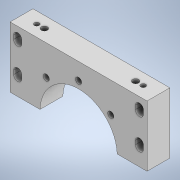
# Autodesk Inventor part: ShooterSeperableClampA
Saved by Autodesk Inventor 2020 (Build 240168000, 168)
## iProperties
Created: 2020-01-29
Part Number: ShooterSeperableClampA
Material: Generic
Document SubType Name: Modeling
Designer: srini
Density: 1 g/cm^3
Appearance: Default
Author: srini
Autodesk Inventor part; units mm, degrees
ref_plane "YZ Plane" through (0, 0, 0) normal (1, 0, 0) x (0, 1, 0)
ref_plane "XZ Plane" through (0, 0, 0) normal (0, 1, 0) x (-1, 0, 0)
ref_plane "XY Plane" through (0, 0, 0) normal (0, 0, 1) x (1, 0, 0)
sketch "Sketch1" plane through (0, 0, 0) normal (0, 0, 1) x (1, 0, 0)
  line L0 (57.15, -25.4) -> (-57.15, -25.4)
  line L1 (-57.15, -25.4) -> (-57.15, 25.4)
  line L2 (-57.15, 25.4) -> (57.15, 25.4)
  line L3 (57.15, 25.4) -> (57.15, -25.4)
  line L4 (57.15, -25.4) -> (-57.15, 25.4) construction
  line L5 (-57.15, -25.4) -> (57.15, 25.4) construction
  point P0 (0, 0)
  point P1 (0, 0)
  point P2 (0, 0)
  dimension "d0" = 114.3
  dimension "d1" = 50.8
  constraints: 12 end point, 3 midpoint, 2 parallel, 1 coincident, 1 horizontal, 1 perpendicular
  measures "d0" distance of L1.end L2.end
  measures "d1" distance of L0.end L1.end
extrude "Extrusion1" add sketch "Sketch1" along normal blind 19.05
sketch "Sketch2" plane through (0, 0, 19.05) normal (0, 0, 1) x (1, 0, 0)
  circle A0 centre (0, -26.67) radius 32.258
  line L0 (-57.15, -25.4) -> (57.15, -25.4) projected
  point P0 (0, 0)
  dimension "d4" = 64.516
  dimension "d6" = 1.27
  constraints: 1 centre point, 1 vertical alignment
  measures "d4" diameter of A0
  measures "d6" distance from line of L0 A0.centre
extrude "Extrusion2" cut sketch "Sketch2" against normal through all
sketch "Sketch3" plane through (0, 0, 19.05) normal (0, 0, 1) x (1, 0, 0)
  line L0 (57.15, 25.4) -> (-57.15, 25.4) projected
  line L1 (-50.8, 14.2875) -> (-50.8, 17.4625) construction
  line L2 (-47.4266, 14.2875) -> (-47.4266, 17.4625)
  line L3 (-54.1734, 17.4625) -> (-54.1734, 14.2875)
  arc A0 (-54.1734, 14.2875) -> (-47.4266, 14.2875) centre (-50.8, 14.2875) ccw
  arc A1 (-47.4266, 17.4625) -> (-54.1734, 17.4625) centre (-50.8, 17.4625) ccw
  line L4 (50.8, 14.2875) -> (50.8, 17.4625) construction
  line L5 (54.1734, 14.2875) -> (54.1734, 17.4625)
  line L6 (47.4266, 17.4625) -> (47.4266, 14.2875)
  arc A2 (47.4266, 14.2875) -> (54.1734, 14.2875) centre (50.8, 14.2875) ccw
  arc A3 (54.1734, 17.4625) -> (47.4266, 17.4625) centre (50.8, 17.4625) ccw
  line L7 (-50.8, -11.1125) -> (-50.8, -7.9375) construction
  line L8 (-47.4266, -11.1125) -> (-47.4266, -7.9375)
  line L9 (-54.1734, -7.9375) -> (-54.1734, -11.1125)
  arc A4 (-54.1734, -11.1125) -> (-47.4266, -11.1125) centre (-50.8, -11.1125) ccw
  arc A5 (-47.4266, -7.9375) -> (-54.1734, -7.9375) centre (-50.8, -7.9375) ccw
  line L10 (50.8, -11.1125) -> (50.8, -7.9375) construction
  line L11 (54.1734, -11.1125) -> (54.1734, -7.9375)
  line L12 (47.4266, -7.9375) -> (47.4266, -11.1125)
  arc A6 (47.4266, -11.1125) -> (54.1734, -11.1125) centre (50.8, -11.1125) ccw
  arc A7 (54.1734, -7.9375) -> (47.4266, -7.9375) centre (50.8, -7.9375) ccw
  point P0 (0, 0)
  point P1 (-50.8, 15.875)
  point P2 (50.8, 15.875)
  point P3 (-50.8, -9.525)
  point P4 (50.8, -9.525)
  dimension "d13" = 3.3734
  dimension "d14" = 3.175
  dimension "d15" = 50.8
  dimension "d16" = 9.525
  dimension "d19" = 101.6
  dimension "d22" = 25.4
  constraints: 32 end point, 16 point on circle, 8 centre point, 4 tangent, 2 vertical, 1 collinear, 1 horizontal, 1 midpoint, 1 parallel, 35 other
  measures "d13" radius of A1
  measures "d14" distance of L1.start L1.end
  measures "d15" distance from line of L1 point (0, 0)
  measures "d16" distance from line of point (-50.8, 15.875) L0
  measures "d19" distance of L2.start L5.start
  measures "d22" distance of L2.start L8.start
extrude "Extrusion3" cut sketch "Sketch3" against normal through all
sketch "Sketch4" plane through (-57.15, 25.4, 0) normal (0, 1, 0) x (1, 0, 0)
  circle A0 centre (19.05, -9.525) radius 2.5797
  circle A1 centre (95.25, -9.525) radius 2.5797
  line L0 (114.3, 0) -> (0, 0) projected
  point P0 (57.15, 0)
  dimension "d27" = 5.1594
  dimension "d28" = 9.525
  dimension "d29" = 38.1
  dimension "d30" = 38.1
  constraints: 2 centre point, 1 equal radius, 1 horizontal alignment
  measures "d27" diameter of A0
  measures "d28" distance from line of A0.centre L0
  measures "d29" horizontal distance of A0.centre point (57.15, 0)
  measures "d30" horizontal distance of A1.centre point (57.15, 0)
extrude "Extrusion4" cut sketch "Sketch4" against normal through all
sketch "Sketch5" plane through (-57.15, -25.4, 0) normal (0, -1, 0) x (1, 0, 0)
  circle A0 centre (12.7, 9.525) radius 2.0193
  circle A1 centre (101.6, 9.525) radius 2.0193
  line L0 (0, 0) -> (24.917, 0) projected
  point P0 (57.15, 0)
  dimension "d33" = 9.525
  dimension "d34" = 4.0386
  dimension "d35" = 44.45
  dimension "d36" = 44.45
  constraints: 2 centre point, 1 equal radius, 1 horizontal alignment
  measures "d33" distance from line of A0.centre L0
  measures "d34" diameter of A0
  measures "d35" horizontal distance of A0.centre point (57.15, 0)
  measures "d36" horizontal distance of A1.centre point (57.15, 0)
extrude "Extrusion5" cut sketch "Sketch5" against normal through all
sketch "Sketch6" plane through (0, 0, 19.05) normal (0, 0, 1) x (1, 0, 0)
  circle A0 centre (-26.9408, 0.2708) radius 2.5797
  arc A1 (32.233, -25.4) -> (-32.233, -25.4) centre (0, -26.67) ccw projected
  circle A2 centre (0, 11.43) radius 2.5797
  circle A3 centre (26.9408, 0.2708) radius 2.5797
  point P0 (0, 0)
  dimension "d39" = 38.1
  dimension "d40" = 5.1594
  dimension "d41" = 45
  dimension "d44" = 90
  constraints: 3 centre point, 5 other
  measures "d39" distance of A0.centre A1.centre
  measures "d40" diameter of A0
extrude "Extrusion6" cut sketch "Sketch6" against normal through all
equation "\"d30\" = d29"
equation "\"d36\" = d35"
body "Solid1"
